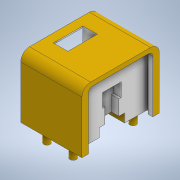
# Autodesk Inventor part: 1D fingertip skeleton new
Saved by Autodesk Inventor 2020 (Build 240168000, 168)
## iProperties
Created: 2020-01-28
Part Number: 1D fingertip skeleton new
Material: Generic
Document SubType Name: Modeling
Designer: kaipa
Density: 1 g/cm^3
Appearance: Default
Author: kaipa
Autodesk Inventor part; units mm, degrees
ref_plane "YZ Plane" through (0, 0, 0) normal (1, 0, 0) x (0, 1, 0)
ref_plane "XZ Plane" through (0, 0, 0) normal (0, 1, 0) x (-1, 0, 0)
ref_plane "XY Plane" through (0, 0, 0) normal (0, 0, 1) x (1, 0, 0)
sketch "Sketch1" plane through (0, 0, 0) normal (1, 0, 0) x (0, 1, 0)
  point P0 (0, 0)
sketch "Sketch2" plane through (0, 0, 0) normal (1, 0, 0) x (0, 1, 0)
  line L0 (7, 8.85) -> (-7, 8.85)
  line L1 (-7, 8.85) -> (-7, -8.85)
  line L2 (-7, -8.85) -> (7, -8.85)
  line L3 (7, -8.85) -> (7, 8.85)
  point P0 (0, 0)
  dimension "d0" = 17.7
  dimension "d1" = 14
  dimension "d2" = 8.85
  dimension "d3" = 7
  constraints: 8 end point, 2 parallel, 1 horizontal, 1 perpendicular
  measures "d0" distance of L0.end L1.end
  measures "d1" distance of L1.end L2.end
  measures "d2" distance from line of point (0, 0) L2
  measures "d3" distance from line of point (0, 0) L1
extrude "Extrusion1" add sketch "Sketch2" along normal blind 14
fillet "Fillet1" radius 2 2 edges at (7, 7, 8.85) (7, 7, -8.85)
sketch "Sketch5" plane through (14, 0, 0) normal (1, 0, 0) x (0, 0, -1)
  line L0 (-7.35, 6) -> (7.35, 6)
  line L1 (7.35, 6) -> (7.35, -7)
  line L2 (7.35, -7) -> (-7.35, -7)
  line L3 (-7.35, -7) -> (-7.35, 6)
  line L4 (6.85, 7) -> (-6.85, 7) projected
  line L5 (8.85, -7) -> (8.85, 5) projected
  line L6 (-8.85, -7) -> (8.85, -7) projected
  line L7 (-8.85, 5) -> (-8.85, -7) projected
  point P0 (0, 0)
  dimension "d19" = 1
  dimension "d20" = 1.5
  dimension "d21" = 0
  dimension "d22" = 1.5
  constraints: 8 end point, 2 parallel, 1 horizontal, 1 perpendicular
  measures "d19" distance between parallel lines of L4 L0
  measures "d20" distance between parallel lines of L5 L1
  measures "d21" distance between parallel lines of L6 L2
  measures "d22" distance between parallel lines of L7 L3
extrude "Extrusion2" cut sketch "Sketch5" against normal blind 2
fillet "Fillet2" radius 1 1 edges at (13, 6, 7.35)
fillet "Fillet3" radius 1 1 edges at (13, 6, -7.35)
ref_plane "Work Plane2" through (7, 0, 0) normal (1, 0, 0) x (0, 0, -1)
mirror "Mirror1" about plane through (7, 0, 0) normal (1, 0, 0) of "Extrusion2"
sketch "Sketch11" plane through (2, -7, -7.35) normal (-1, 0, 0) x (0, 0, 1)
  line L0 (4.45, 2) -> (10.25, 2)
  line L1 (10.25, 2) -> (10.25, 6.7)
  line L2 (10.25, 6.7) -> (4.45, 6.7)
  line L3 (4.45, 6.7) -> (4.45, 2)
  line L4 (10.725, 6.7) -> (3.975, 6.7)
  line L5 (3.975, 6.7) -> (3.975, 10)
  line L6 (3.975, 10) -> (10.725, 10)
  line L7 (10.725, 10) -> (10.725, 6.7)
  line L8 (14.7, 0) -> (0, 0) projected
  point P0 (7.35, 7)
  point P1 (10.25, 6.7)
  dimension "d52" = 5.8
  dimension "d53" = 4.7
  dimension "d54" = 2
  dimension "d55" = 3.3
  dimension "d56" = 6.75
  dimension "d57" = 2.9
  dimension "d58" = 3.375
  constraints: 16 end point, 4 parallel, 2 horizontal, 2 perpendicular, 1 collinear
  measures "d52" distance of L0.start L0.end
  measures "d53" distance of L2.end L0.start
  measures "d54" distance between parallel lines of L8 L0
  measures "d55" distance of L4.end L5.end
  measures "d56" distance of L5.end L6.end
  measures "d57" distance from line of point (7.35, 7) L3
  measures "d58" distance from line of point (7.35, 7) L5
extrude "Extrusion5" cut sketch "Sketch11" against normal blind 3.3
fillet "Fillet4" radius 0.001 2 edges at (3.65, 3, -3.375) (3.65, 3, 3.375)
fillet "Fillet5" radius 0.001 2 edges at (3.65, -0.3, -3.375) (3.65, -0.3, 3.375)
fillet "Fillet6" radius 1 1 edges at (1, 6, 7.35)
fillet "Fillet7" radius 1 1 edges at (1, 6, -7.35)
sketch "Sketch15" plane through (0, -7, -8.85) normal (0, -1, 0) x (1, 0, 0)
  line L0 (0, 2) -> (14, 2) projected
  circle A0 centre (4, 2) radius 0.75
  line L1 (0, 1.5) -> (0, 0) projected
  line L2 (12, 1.5) -> (12, 16.2) projected
  line L3 (2, 16.2) -> (2, 1.5) projected
  line L4 (7, 21.24) -> (7, -3.54) projected
  point P0 (0, 8.85)
  point P1 (12, 3.75)
  point P2 (2, 3.35)
  dimension "d74" = 1.5
  dimension "d120" = 4
  constraints: 1 centre point, 1 point on line
  measures "d74" diameter of A0
  measures "d120" distance from line of L1 A0.centre
sketch "Sketch15 outline for Extrusion8" plane through (0, -7, -8.85) normal (0, -1, 0) x (1, 0, 0)
  circle A0 centre (4, 2) radius 0.75
extrude "Extrusion8" add sketch "Sketch15 outline for Extrusion8" along normal blind 3 draft -0.5
mirror "Mirror3" about plane through (0, 0, 0) normal (0, 0, 1) of "Extrusion8"
mirror "Mirror4" about plane through (7, 0, 0) normal (1, 0, 0) of "Extrusion8", "Mirror3"
sketch "Sketch18" plane through (2, 3, -3.374) normal (0, -1, 0) x (1, 0, 0)
  line L0 (3.3, -0.001) -> (0, -0.001)
  line L1 (0, -0.001) -> (0, 6.749)
  line L2 (0, 6.749) -> (3.3, 6.749)
  line L3 (3.3, 6.749) -> (3.3, -0.001)
  line L4 (0, -0.001) -> (3.3, -0.001) projected
  line L5 (3.3, 6.749) -> (0, 6.749) projected
  line L6 (0, 0) -> (0, 6.748) projected
  line L7 (3.3, 0) -> (3.3, 6.748) projected
  point P0 (-2, 3.374)
  constraints: 8 end point, 4 collinear, 2 parallel, 1 horizontal, 1 perpendicular
extrude "Extrusion9" cut sketch "Sketch18" against normal through all
sketch "Sketch19" plane through (0, -7, 8.85) normal (0, -1, 0) x (1, 0, 0)
  line L0 (13, -0.8) -> (12, -0.8)
  line L1 (12, -0.8) -> (12, -1.5)
  line L2 (12, -1.5) -> (13, -1.5)
  line L3 (13, -1.5) -> (13, -0.8)
  point P0 (0, -8.85)
  dimension "d103" = 0.7
  dimension "d104" = 1
  constraints: 8 end point, 2 parallel, 1 horizontal, 1 perpendicular
  measures "d103" distance of L0.end L1.end
  measures "d104" distance of L0.start L0.end
sketch3d "3D Sketch3"
  line L0 (14, -7, 7.35) -> (14, 5, 7.35)
  arc A0 (14, 5, 7.35) -> (14, 6, 6.35) centre (14, 5, 6.35) ccw
  line L1 (14, 6, 6.35) -> (14, 6, -6.35)
  arc A1 (14, 6, -6.35) -> (14, 5, -7.35) centre (14, 5, -6.35) ccw
  line L2 (14, 5, -7.35) -> (14, -7, -7.35)
sweep "Sweep3" cut profiles "Sketch19" path "3D Sketch3"
mirror "Mirror6" about plane through (7, 0, 0) normal (1, 0, 0) of "Sweep3"
sketch "Sketch20" plane through (12, 0, 0) normal (1, 0, 0) x (0, 0, -1)
  line L0 (-2.9, -5) -> (2.9, -5)
  line L1 (2.9, -5) -> (2.9, -7)
  line L2 (2.9, -7) -> (-2.9, -7)
  line L3 (-2.9, -7) -> (-2.9, -5)
  line L4 (3.6, 4.6) -> (3.6, -4.3)
  line L5 (-3.6, -4.3) -> (-3.6, 5.3)
  line L6 (3.6, -4.3) -> (-3.6, -4.3)
  line L7 (5.45, -7) -> (-5.45, -7)
  point P0 (0, 0)
  dimension "d109" = 0.7
  dimension "d110" = 0.7
  dimension "d116" = 2
  constraints: 16 end point
  measures "d109" distance between parallel lines of L4 L1
  measures "d110" distance between parallel lines of L5 L3
  measures "d116" distance of L0.end L1.end
extrude "Extrusion10" cut sketch "Sketch20" against normal through all
sketch "Sketch22" plane through (12, 0, 0) normal (1, 0, 0) x (0, 0, -1)
  line L0 (-2.11, 1.56) -> (2.11, 1.56)
  line L1 (2.11, 1.56) -> (2.11, -1.56)
  line L2 (2.11, -1.56) -> (-2.11, -1.56)
  line L3 (-2.11, -1.56) -> (-2.11, 1.56)
  line L4 (-1.61, -1.56) -> (1.61, -1.56)
  line L5 (1.61, -1.56) -> (1.61, -5)
  line L6 (1.61, -5) -> (-1.61, -5)
  line L7 (-1.61, -5) -> (-1.61, -1.56)
  line L8 (-2.9, -5) -> (2.9, -5) projected
  point P0 (0, 0)
  dimension "d121" = 4.22
  dimension "d122" = 3.12
  dimension "d123" = 2.11
  dimension "d124" = 1.56
  dimension "d125" = 3.22
  dimension "d126" = 1.61
  constraints: 16 end point, 4 parallel, 2 collinear, 2 horizontal, 2 perpendicular
  measures "d121" distance of L0.start L0.end
  measures "d122" distance of L0.end L1.end
  measures "d123" distance from line of point (0, 0) L1
  measures "d124" distance from line of point (0, 0) L2
  measures "d125" distance between parallel lines of L5 L7
  measures "d126" distance from line of point (0, 0) L5
extrude "Extrusion12" cut sketch "Sketch22" against normal blind 1.72
equation "\"d2\" = 0.5 * d0"
equation "\"d3\" = 0.5 * d1"
equation "\"d57\" = 0.5 * d52"
equation "\"d58\" = 0.5 * d56"
equation "\"d123\" = 0.5 * d121"
equation "\"d124\" = 0.5 * d122"
equation "\"d126\" = 0.5 * d125"
body "Solid1"
